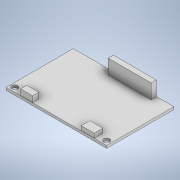
# Autodesk Inventor part: XDSEmulatorModule
Saved by Autodesk Inventor 2022.2 (Build 262287000, 287)
## iProperties
Created: 2022-01-14
Part Number: XDSEmulatorModule
Material: Generic
Document SubType Name: Modeling
Designer: Max
Density: 1 g/cm^3
Appearance: Default
Author: Max
Autodesk Inventor part; units mm, degrees
ref_plane "YZ Plane" through (0, 0, 0) normal (1, 0, 0) x (0, 1, 0)
ref_plane "XZ Plane" through (0, 0, 0) normal (0, 1, 0) x (-1, 0, 0)
ref_plane "XY Plane" through (0, 0, 0) normal (0, 0, 1) x (1, 0, 0)
sketch "Base Board" plane through (0, 0, 0) normal (0, 1, 0) x (-1, 0, 0)
  line L0 (5.0631, 4.2478) -> (-53.4369, 4.2478)
  line L1 (-53.4369, 4.2478) -> (-53.4369, -34.8522)
  line L2 (-53.4369, -34.8522) -> (5.0631, -34.8522)
  line L3 (5.0631, -34.8522) -> (5.0631, 4.2478)
  circle A0 centre (2.5631, 1.7478) radius 1.755
  circle A1 centre (-50.9369, 1.7478) radius 1.755
  point P0 (0, 0)
  dimension "d0" = 58.5
  dimension "d1" = 39.1
  dimension "d6" = 3.51
  dimension "d8" = 3.51
  dimension "d10" = 2.5
  dimension "d11" = 2.5
  dimension "d12" = 2.5
  dimension "d13" = 2.5
  constraints: 8 end point, 2 centre point, 2 parallel, 1 horizontal, 1 perpendicular
  measures "d0" distance of L2.end L1.end
  measures "d1" distance of L1.end L0.end
  measures "d6" diameter of A0
  measures "d8" diameter of A1
  measures "d10" distance from line of L0 A0.centre
  measures "d11" distance from line of L3 A0.centre
  measures "d12" distance from line of L1 A1.centre
  measures "d13" distance from line of L0 A1.centre
extrude "Base Extrusion" add sketch "Base Board" along normal blind 1.5
sketch "Sketch2" plane through (0, 1.5, 0) normal (0, 1, 0) x (1, 0, 0)
  line L0 (38.5869, -4.1507) -> (46.1869, -4.1507)
  line L1 (46.1869, -4.1507) -> (46.1869, 0.8493)
  line L2 (46.1869, 0.8493) -> (38.5869, 0.8493)
  line L3 (38.5869, 0.8493) -> (38.5869, -4.1507)
  line L4 (-5.0631, 34.8522) -> (-5.0631, -4.2478) projected
  line L5 (53.4369, -4.2478) -> (53.4369, 34.8522) projected
  dimension "d16" = 7.6
  dimension "d17" = 5
  dimension "d21" = 7.25
  constraints: 8 end point, 2 parallel, 1 horizontal, 1 perpendicular
  measures "d16" distance of L2.end L1.end
  measures "d17" distance of L1.end L0.end
  measures "d21" distance between parallel lines of L5 L1
extrude "MicroUSB slot" add sketch "Sketch2" along normal blind 2.5
sketch "Sketch3" plane through (0, 1.5, 0) normal (0, 1, 0) x (1, 0, 0)
  line L0 (3.2869, -4.0967) -> (10.2869, -4.0967)
  line L1 (10.2869, -4.0967) -> (10.2869, -0.5967)
  line L2 (10.2869, -0.5967) -> (3.2869, -0.5967)
  line L3 (3.2869, -0.5967) -> (3.2869, -4.0967)
  line L4 (-5.0631, 34.8522) -> (-5.0631, -4.2478) projected
  point P0 (0, 0)
  dimension "d22" = 7
  dimension "d23" = 3.5
  dimension "d24" = 8.35
  constraints: 8 end point, 2 parallel, 1 horizontal, 1 perpendicular
  measures "d22" distance of L2.end L1.end
  measures "d23" distance of L1.end L0.end
  measures "d24" distance between parallel lines of L4 L3
extrude "Reset Button" add sketch "Sketch3" along normal blind 3.35
sketch "Sketch4" plane through (0, 1.5, 0) normal (0, 1, 0) x (1, 0, 0)
  line L0 (43.4369, 31.6613) -> (18.4369, 31.6613)
  line L1 (18.4369, 31.6613) -> (18.4369, 34.6613)
  line L2 (18.4369, 34.6613) -> (43.4369, 34.6613)
  line L3 (43.4369, 34.6613) -> (43.4369, 31.6613)
  line L4 (53.4369, -4.2478) -> (53.4369, 34.8522) projected
  point P0 (0, 0)
  point P1 (43.4369, 33.1613)
  dimension "d27" = 25
  dimension "d28" = 3
  dimension "d29" = 10
  constraints: 8 end point, 2 parallel, 1 horizontal, 1 midpoint, 1 perpendicular
  measures "d27" distance of L1.end L2.end
  measures "d28" distance of L0.end L1.end
  measures "d29" distance from line of L4 point (43.437, 33.161)
extrude "Extrusion4" add sketch "Sketch4" along normal blind 8.55
body "Solid1"
